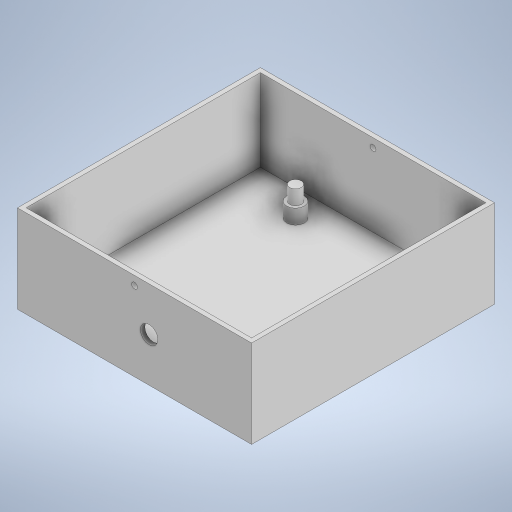
# Autodesk Inventor part: Gyrosensor
Saved by Autodesk Inventor 2024 (Build 280153000, 153)
## iProperties
Created: 2024-01-17
Part Number: Gyrosensor
Material: Generisch
Document SubType Name: Modeling
Designer: User
Density: 1 g/cm^3
Appearance: Vorgabe
Author: User
Autodesk Inventor part; units mm, degrees
ref_plane "YZ Plane" through (0, 0, 0) normal (1, 0, 0) x (0, 1, 0)
ref_plane "XZ Plane" through (0, 0, 0) normal (0, 1, 0) x (-1, 0, 0)
ref_plane "XY Plane" through (0, 0, 0) normal (0, 0, 1) x (1, 0, 0)
sketch "Skizze1" plane through (0, 0, 0) normal (0, 0, 1) x (1, 0, 0)
  line L0 (0, 0) -> (80, 0)
  line L1 (80, 0) -> (80, 83)
  line L2 (80, 83) -> (0, 83)
  line L3 (0, 83) -> (0, 0)
  line L4 (1.5, 81.5) -> (78.5, 81.5)
  line L5 (78.5, 81.5) -> (78.5, 1.5)
  line L6 (78.5, 1.5) -> (1.5, 1.5)
  line L7 (1.5, 1.5) -> (1.5, 81.5)
  dimension "d0" = 80
  dimension "d1" = 83
  dimension "d2" = 1.5
  dimension "d3" = 1.5
  dimension "d4" = 1.5
  dimension "d5" = 1.5
  constraints: 16 end point, 4 parallel, 2 horizontal, 2 perpendicular
  measures "d0" distance of L2.end L1.end
  measures "d1" distance of L1.end L0.end
  measures "d2" distance between parallel lines of L2 L4
  measures "d3" distance between parallel lines of L3 L7
  measures "d4" distance between parallel lines of L0 L6
  measures "d5" distance between parallel lines of L1 L5
extrude "Extrusion1" add sketch "Skizze1" along normal blind 2 contours L4 L5 L6 L7
extrude "Extrusion2" add sketch "Skizze1" along normal blind 30
sketch "Skizze2" plane through (0, 0, 2) normal (0, 0, 1) x (1, 0, 0)
  circle A0 centre (22.5, 72.5) radius 3
  circle A1 centre (21, 10.5) radius 3
  line L0 (1.5, 1.5) -> (1.5, 81.5) projected
  circle A2 centre (22.5, 72.5) radius 2
  circle A3 centre (21, 10.5) radius 2
  circle A4 centre (65.5, 41.5) radius 1
  circle A5 centre (65.5, 41.5) radius 2.5
  line L1 (78.5, 81.5) -> (78.5, 1.5) projected
  line L2 (78.5, 1.5) -> (1.5, 1.5) projected
  line L3 (1.5, 81.5) -> (78.5, 81.5) projected
  point P0 (0, 0)
  dimension "d11" = 21
  dimension "d12" = 19.5
  dimension "d13" = 4
  dimension "d14" = 4
  dimension "d15" = 6
  dimension "d16" = 6
  dimension "d17" = 2
  dimension "d18" = 5
  dimension "d23" = 13
  dimension "d31" = 62
  dimension "d32" = 9
  dimension "d33" = 9
  constraints: 6 centre point, 3 coincident
  measures "d11" distance from line of L0 A0.centre
  measures "d12" distance from line of L0 A1.centre
  measures "d13" diameter of A2
  measures "d14" diameter of A3
  measures "d15" diameter of A0
  measures "d16" diameter of A1
  measures "d17" diameter of A4
  measures "d18" diameter of A5
  measures "d23" distance from line of A4.centre L1
  measures "d31" vertical distance of A1.centre A0.centre
  measures "d32" distance from line of L2 A1.centre
  measures "d33" distance from line of L3 A0.centre
extrude "Extrusion3" add sketch "Skizze2" along normal blind 5 contours A0 | A1 | A5
extrude "Extrusion4" add sketch "Skizze2" along normal blind 10 contours A2 | A3
sketch "Skizze4" plane through (0, 0, 0) normal (0, -1, 0) x (1, 0, 0)
  circle A0 centre (40, 27) radius 1
  line L0 (0, 30) -> (80, 30) projected
  line L1 (0, 0) -> (0, 30) projected
  dimension "d34" = 2
  dimension "d35" = 3
  dimension "d36" = 40
  constraints: 1 centre point
  measures "d34" diameter of A0
  measures "d35" distance from line of L0 A0.centre
  measures "d36" distance from line of L1 A0.centre
extrude "Extrusion6" cut sketch "Skizze4" against normal through all
sketch "Skizze5" plane through (0, 0, 0) normal (0, -1, 0) x (1, 0, 0)
  circle A0 centre (45, 15) radius 3
  line L0 (0, 0) -> (0, 30) projected
  line L1 (0, 30) -> (80, 30) projected
  dimension "d39" = 6
  dimension "d40" = 45
  dimension "d41" = 15
  constraints: 1 centre point
  measures "d39" diameter of A0
  measures "d40" distance from line of L0 A0.centre
  measures "d41" distance from line of L1 A0.centre
extrude "Extrusion7" cut sketch "Skizze5" against normal blind 5
